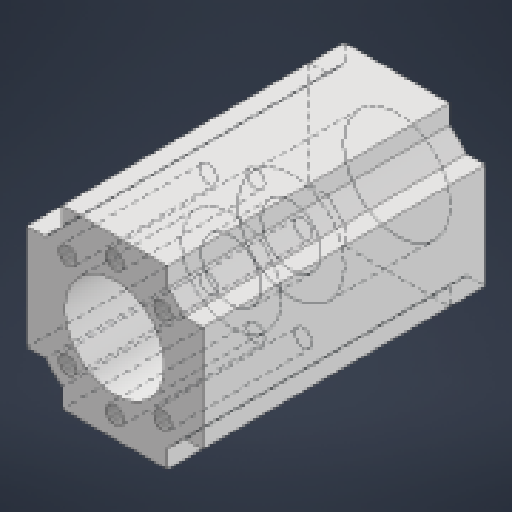
# Autodesk Inventor part: SLIDER_80
Saved by Autodesk Inventor 2023 (Build 270158000, 158)
## iProperties
Created: 2025-09-04
Part Number: SLIDER_80
Material: 일반
Document SubType Name: Modeling
Designer: k
Density: 1 g/cm^3
Appearance: 기본값
Author: k
Autodesk Inventor part; units mm, degrees
ref_plane "YZ Plane" through (0, 0, 0) normal (1, 0, 0) x (0, 1, 0)
ref_plane "XZ Plane" through (0, 0, 0) normal (0, 1, 0) x (-1, 0, 0)
ref_plane "XY Plane" through (0, 0, 0) normal (0, 0, 1) x (1, 0, 0)
sketch "스케치2" plane through (0, 0, 0) normal (0, 0, 1) x (1, 0, 0)
  circle A0 centre (143.202, -118.4807) radius 24.65
  line L0 (118.202, -93.4807) -> (168.202, -93.4807)
  line L1 (168.202, -93.4807) -> (168.202, -143.4807)
  line L2 (168.202, -143.4807) -> (118.202, -143.4807)
  line L3 (118.202, -143.4807) -> (118.202, -93.4807)
  line L4 (158.102, -143.4807) -> (158.102, -93.4807)
  line L5 (168.202, -103.5807) -> (118.202, -103.5807)
  line L6 (128.302, -93.4807) -> (128.302, -143.4807)
  line L7 (118.202, -133.3807) -> (168.202, -133.3807)
  point P0 (0, 0)
  point P1 (128.302, -98.8437)
  point P2 (123.565, -103.5807)
  point P3 (123.565, -133.3807)
  point P4 (128.302, -138.1178)
  point P5 (158.102, -138.1178)
  point P6 (162.839, -133.3807)
  point P7 (162.839, -103.5807)
  point P8 (158.102, -98.8437)
  dimension "d13" = 49.3
  dimension "d15" = 50
  dimension "d17" = 25
  dimension "d19" = 29.8
  dimension "d20" = 50
  dimension "d21" = 25
  dimension "d23" = 14.9
  dimension "d24" = 14.9
  dimension "d25" = 29.8
  constraints: 16 end point, 8 point on line, 4 parallel, 2 perpendicular, 1 centre point, 1 horizontal
  measures "d13" diameter of A0
  measures "d15" distance of L0.end L1.end
  measures "d17" distance from line of L1 A0.centre
  measures "d19" distance between parallel lines of L6 L4
  measures "d20" distance between parallel lines of L1 L3
  measures "d21" distance from line of A0.centre L0
  measures "d23" distance from line of A0.centre L4
  measures "d24" distance from line of A0.centre L5
  measures "d25" distance between parallel lines of L7 L5
extrude "돌출2" add sketch "스케치2" along normal blind 80 contours A0 L7 L4 L5 | A0 L5 L1 L7 | L5 L4 A0 | A0 L4 L7 | L4 L5 L6 A0 | A0 L6 L0 L4 | L4 L7 L6 L5 | L4 L2 L6 A0 | A0 L6 L7 L4 | L6 L5 A0 | L6 L7 A0 L5 | A0 L7 L6 | A0 L7 L3 L5
sketch "스케치3" plane through (0, 0, 80) normal (0, 0, 1) x (1, 0, 0)
  arc A0 (162.839, -103.5807) -> (158.102, -98.8437) centre (143.202, -118.4807) ccw projected
  circle A1 centre (143.202, -118.4807) radius 14.1
  point P0 (0, 0)
  dimension "d28" = 28.2
  constraints: 1 centre point, 1 coincident
  measures "d28" diameter of A1
extrude "돌출3" cut sketch "스케치3" against normal blind 33
sketch "스케치4" plane through (0, 0, 0) normal (0, 0, -1) x (-1, 0, 0)
  arc A0 (-128.302, -138.1178) -> (-123.565, -133.3807) centre (-143.202, -118.4807) ccw projected
  circle A1 centre (-143.202, -118.4807) radius 15.1
  point P0 (0, 0)
  dimension "d31" = 30.2
  constraints: 1 centre point, 1 coincident
  measures "d31" diameter of A1
extrude "돌출4" cut sketch "스케치4" against normal blind 30
sketch "스케치5" plane through (0, 0, 80) normal (0, 0, 1) x (1, 0, 0)
  circle A0 centre (143.202, -118.4807) radius 14.1 projected
  circle A1 centre (143.202, -118.4807) radius 8.5
  point P0 (0, 0)
  dimension "d34" = 17
  constraints: 1 centre point, 1 coincident
  measures "d34" diameter of A1
extrude "돌출5" cut sketch "스케치5" against normal through all contours A1
sketch "스케치6" plane through (0, 0, 80) normal (0, 0, 1) x (1, 0, 0)
  circle A0 centre (143.202, -118.4807) radius 8.5 projected
  circle A1 centre (143.202, -118.4807) radius 19
  circle A2 centre (143.202, -99.4807) radius 2.5
  line L0 (143.202, -118.4807) -> (178.3285, -118.4807) construction
  circle A3 centre (129.767, -105.0457) radius 2.5
  line L1 (143.202, -118.4807) -> (143.202, -86.2769)
  line L2 (143.202, -118.4807) -> (175.4059, -118.4807) construction
  circle A4 centre (156.637, -105.0457) radius 2.5
  circle A5 centre (143.202, -137.4807) radius 2.5
  circle A6 centre (129.767, -131.9158) radius 2.5
  circle A7 centre (156.637, -131.9158) radius 2.5
  point P0 (0, 0)
  dimension "d37" = 38
  dimension "d38" = 5
  dimension "d44" = 45
  dimension "d46" = 90
  constraints: 6 centre point, 6 end point, 4 symmetric about line, 2 horizontal, 1 coincident, 1 perpendicular, 1 vertical alignment, 9 other
  measures "d38" diameter of A2
  measures "d46" angle of L2 L1
extrude "돌출6" cut sketch "스케치6" against normal blind 40 contours A4 A1 | A1 A4 | A7 A1 | A1 A7 | A2 L1 A1 | A1 L1 A2 | A5 A1 | A1 A5 | L1 A2 A1 | A1 A2 L1 | A6 A1 | A1 A6 | A3 A1 | A1 A3
thread "스레드1" size "M5x0.8" class "6H" standard "ANSI Metric M Profile" full length
thread "스레드2" size "M5x0.8" class "6H" standard "ANSI Metric M Profile" full length
thread "스레드3" size "M5x0.8" class "6H" standard "ANSI Metric M Profile" full length
thread "스레드4" size "M5x0.8" class "6H" standard "ANSI Metric M Profile" full length
thread "스레드5" size "M5x0.8" class "6H" standard "ANSI Metric M Profile" full length
thread "스레드6" size "M5x0.8" class "6H" standard "ANSI Metric M Profile" full length
